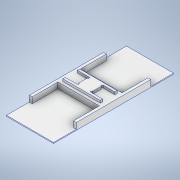
# Autodesk Inventor part: Niz_Plita
Saved by Autodesk Inventor 2020.1 (Build 241239000, 239)
## iProperties
Created: 2023-01-07
Part Number: Niz_Plita
Material: Алюминий 6061
Document SubType Name: Modeling
Designer: KirikDK
Density: 2.7 g/cm^3
Appearance: Алюминий — плоский
Mass: 2934.89 g
Surface Area: 2557.51 cm^2
Volume: 1086.99 cm^3
Author: KirikDK
Autodesk Inventor part; units mm, degrees
ref_plane "YZ Plane" through (0, 0, 0) normal (1, 0, 0) x (0, 1, 0)
ref_plane "XZ Plane" through (0, 0, 0) normal (0, 1, 0) x (-1, 0, 0)
ref_plane "XY Plane" through (0, 0, 0) normal (0, 0, 1) x (1, 0, 0)
sketch "Эскиз1" plane through (0, 0, 0) normal (1, 0, 0) x (0, 1, 0)
  line L0 (29, 218.9091) -> (0, 218.9091)
  line L1 (0, 218.9091) -> (0, -297.0909)
  line L2 (0, -297.0909) -> (29, -297.0909)
  line L3 (29, -297.0909) -> (29, 218.9091)
  point P0 (0, 0)
  dimension "d0" = 516
  dimension "d1" = 29
  constraints: 8 end point, 2 parallel, 1 horizontal, 1 perpendicular
  measures "d0" distance of L0.end L1.end
  measures "d1" distance of L0.start L0.end
extrude "Выдавливание1" add sketch "Эскиз1" along normal blind 200
sketch "Эскиз2" plane through (0, 29, 218.9091) normal (0, 1, 0) x (1, 0, 0)
  line L0 (0, 516) -> (0, 0) projected
  line L1 (0, 0) -> (200, 0) projected
  line L2 (200, 516) -> (200, 0) projected
  line L3 (0, 516) -> (200, 516) projected
  line L4 (20, 232) -> (180, 232)
  line L5 (180, 232) -> (180, 284)
  line L6 (180, 284) -> (20, 284)
  line L7 (20, 284) -> (20, 232)
  line L8 (20, 232) -> (180, 232)
  line L9 (180, 232) -> (180, 222)
  line L10 (180, 222) -> (20, 222)
  line L11 (20, 222) -> (20, 232)
  line L12 (20, 284) -> (180, 284)
  line L13 (180, 284) -> (180, 294)
  line L14 (180, 294) -> (20, 294)
  line L15 (20, 294) -> (20, 284)
  line L16 (70, 232) -> (130, 232)
  line L17 (130, 232) -> (130, 284)
  line L18 (130, 284) -> (70, 284)
  line L19 (70, 284) -> (70, 232)
  circle A0 centre (70, 236) radius 4
  circle A1 centre (70, 280) radius 4
  circle A2 centre (130, 280) radius 4
  circle A3 centre (130, 236) radius 4
  point P0 (0, 218.9091)
  point P1 (130, 240)
  point P2 (130, 276)
  point P3 (70, 276)
  point P4 (70, 240)
  dimension "d4" = 52
  dimension "d5" = 20
  dimension "d6" = 20
  dimension "d7" = 232
  dimension "d8" = 232
  dimension "d9" = 10
  dimension "d10" = 10
  dimension "d11" = 50
  dimension "d12" = 50
  constraints: 32 end point, 8 parallel, 7 point on line, 4 horizontal, 4 perpendicular, 12 other
  measures "d4" distance of L6.end L4.start
  measures "d5" distance between parallel lines of L0 L7
  measures "d6" distance between parallel lines of L2 L5
  measures "d7" distance between parallel lines of L1 L4
  measures "d8" distance between parallel lines of L3 L6
  measures "d9" distance between parallel lines of L10 L4
  measures "d10" distance between parallel lines of L14 L6
  measures "d11" distance between parallel lines of L7 L19
  measures "d12" distance between parallel lines of L5 L17
extrude "Выдавливание2" add sketch "Эскиз2" along normal blind 10 contours L4 L9 L10 L11 | A0 L19 A1 L6 A2 L17 A3 L4 | L15 L14 L13 L6
sketch "Эскиз3" plane through (0, 29, 218.9091) normal (0, 1, 0) x (1, 0, 0)
  line L0 (180, 294) -> (180, 284) projected
  line L1 (180, 284) -> (130, 284) projected
  arc A0 (130, 284) -> (130, 276) centre (130, 280) ccw projected
  line L2 (130, 276) -> (130, 240) projected
  arc A1 (130, 240) -> (130, 232) centre (130, 236) ccw projected
  line L3 (130, 232) -> (180, 232) projected
  line L4 (180, 232) -> (180, 222) projected
  line L5 (180, 222) -> (20, 222) projected
  line L6 (20, 222) -> (20, 232) projected
  line L7 (20, 232) -> (70, 232) projected
  arc A2 (70, 232) -> (70, 240) centre (70, 236) ccw projected
  line L8 (70, 240) -> (70, 276) projected
  arc A3 (70, 276) -> (70, 284) centre (70, 280) ccw projected
  line L9 (70, 284) -> (20, 284) projected
  line L10 (20, 284) -> (20, 294) projected
  line L11 (20, 294) -> (180, 294) projected
  line L12 (0, 516) -> (0, 0) projected
  line L13 (0, 0) -> (200, 0) projected
  line L14 (200, 516) -> (200, 0) projected
  line L15 (0, 516) -> (200, 516) projected
  line L16 (12, 12) -> (12, 504)
  line L17 (12, 504) -> (188, 504)
  line L18 (188, 504) -> (188, 12)
  line L19 (188, 12) -> (12, 12)
  line L20 (8, 210) -> (192, 210)
  line L21 (192, 210) -> (192, 244)
  line L22 (192, 244) -> (142, 244)
  line L23 (142, 244) -> (142, 272)
  line L24 (142, 272) -> (192, 272)
  line L25 (192, 272) -> (192, 306)
  line L26 (192, 306) -> (8, 306)
  line L27 (8, 306) -> (8, 272)
  line L28 (8, 272) -> (58, 272)
  line L29 (58, 272) -> (58, 244)
  line L30 (58, 244) -> (8, 244)
  line L31 (8, 244) -> (8, 210)
  line L32 (-28, 416) -> (286, 416)
  line L33 (286, 416) -> (286, 100)
  line L34 (286, 100) -> (-28, 100)
  line L35 (-28, 100) -> (-28, 416)
  point P0 (0, 218.9091)
  point P1 (0, 416)
  point P2 (12, 416)
  point P3 (12, 306)
  point P4 (188, 306)
  point P5 (188, 416)
  point P6 (200, 416)
  point P7 (200, 100)
  point P8 (188, 100)
  point P9 (188, 210)
  point P10 (12, 210)
  point P11 (12, 100)
  point P12 (0, 100)
  dimension "d15" = 100
  dimension "d16" = 100
  constraints: 40 end point, 2 parallel, 1 horizontal, 1 perpendicular, 14 other
  measures "d15" distance between parallel lines of L15 L32
  measures "d16" distance between parallel lines of L13 L34
extrude "Выдавливание3" cut sketch "Эскиз3" against normal blind 25 contours L15 L14 L32 L18 L17 L16 L12 | L34 L16 L19 L18 L14 L13 L12 | L32 L18 L26 L16 | L16 L17 L18 L32 | L34 L18 L19 L16 | L16 L20 L18 L34
sketch "Эскиз4" plane through (200, 0, 0) normal (1, 0, 0) x (0, 0, -1)
  line L0 (-218.9091, 0) -> (-215.9091, 0)
  line L1 (-215.9091, 0) -> (-215.9091, 13.6393)
  line L2 (-215.9091, 13.6393) -> (-218.9091, 13.6393)
  line L3 (-218.9091, 13.6393) -> (-218.9091, 0)
  line L4 (297.0909, 0) -> (297.0909, 4) projected
  line L5 (297.0909, 0) -> (294.0909, 0)
  line L6 (294.0909, 0) -> (294.0909, 8)
  line L7 (294.0909, 8) -> (297.0909, 8)
  line L8 (297.0909, 8) -> (297.0909, 0)
  point P0 (0, 0)
  dimension "d19" = 3
  dimension "d20" = 3
  constraints: 16 end point, 4 parallel, 2 horizontal, 2 perpendicular
  measures "d19" distance of L0.start L0.end
  measures "d20" distance of L4.start L5.end
extrude "Выдавливание4" cut sketch "Эскиз4" against normal blind 1000
